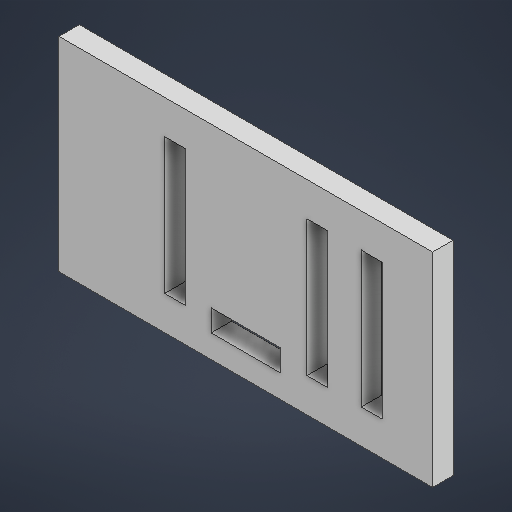
# Autodesk Inventor part: Moving_rail
Saved by Autodesk Inventor 2027 (Build 310192000, 192)
## iProperties
Created: 2026-05-09
Part Number: Moving_rail
Material: Generic
Document SubType Name: Modeling
Designer: alexy
Density: 1 g/cm^3
Appearance: Default
Mass: 3.22008 g
Surface Area: 29.3032 cm^2
Volume: 3.22008 cm^3
Author: alexy
Autodesk Inventor part; units mm, degrees
ref_plane "YZ Plane" through (0, 0, 0) normal (1, 0, 0) x (0, 1, 0)
ref_plane "XZ Plane" through (0, 0, 0) normal (0, 1, 0) x (-1, 0, 0)
ref_plane "XY Plane" through (0, 0, 0) normal (0, 0, 1) x (1, 0, 0)
sketch "Sketch1" plane through (0, 0, 0) normal (0, 0, 1) x (1, 0, 0)
  line L0 (0, 0) -> (55, 0)
  line L1 (55, 0) -> (55, 30)
  line L2 (55, 30) -> (0, 30)
  line L3 (0, 30) -> (0, 0)
  line L4 (36.5, 25) -> (39.55, 25)
  line L5 (39.55, 25) -> (39.55, 5)
  line L6 (39.55, 5) -> (36.5, 5)
  line L7 (36.5, 5) -> (36.5, 25)
  line L8 (15.55, 25) -> (18.6, 25)
  line L9 (18.6, 25) -> (18.6, 5)
  line L10 (18.6, 5) -> (15.55, 5)
  line L11 (15.55, 5) -> (15.55, 25)
  line L12 (44.5, 25) -> (47.55, 25)
  line L13 (47.55, 25) -> (47.55, 5)
  line L14 (47.55, 5) -> (44.5, 5)
  line L15 (44.5, 5) -> (44.5, 25)
  point P0 (15.55, 15)
  point P1 (0, 15)
  point P2 (36.5, 15)
  point P3 (17.075, 5)
  point P4 (27.5, 30)
  dimension "d0" = 55
  dimension "d1" = 30
  dimension "d2" = 3.05
  dimension "d3" = 3.05
  dimension "d4" = 24
  dimension "d6" = 10
  dimension "d7" = 8.9
  dimension "d16" = 3.05
  dimension "d17" = 32
  constraints: 32 end point, 8 parallel, 5 midpoint, 4 horizontal, 4 horizontal alignment, 4 perpendicular, 2 point on line
  measures "d0" distance of L2.end L1.end
  measures "d1" distance of L0.end L1.end
  measures "d2" distance of L5.end L6.end
  measures "d3" distance of L9.end L10.end
  measures "d4" distance between parallel lines of L11 L5
  measures "d6" vertical distance of point (15.55, 15) point (17.075, 5)
  measures "d7" distance from line of L9 point (27.5, 30)
  measures "d16" distance of L13.end L14.end
  measures "d17" distance of L10.end L13.end
extrude "Extrusion1" add sketch "Sketch1" along normal blind 3
sketch "Sketch2" plane through (0, 0, 3) normal (0, 0, 1) x (1, 0, 0)
  line L0 (22.4, 6.6) -> (32.6, 6.6)
  line L1 (32.6, 6.6) -> (32.6, 3.4)
  line L2 (32.6, 3.4) -> (22.4, 3.4)
  line L3 (22.4, 3.4) -> (22.4, 6.6)
  line L4 (22.4, 6.6) -> (32.6, 3.4) construction
  line L5 (32.6, 6.6) -> (22.4, 3.4) construction
  line L6 (55, 30) -> (0, 30) projected
  line L7 (0, 0) -> (55, 0) projected
  point P0 (27.5, 5)
  point P1 (27.5, 30)
  point P2 (27.5, 30)
  dimension "d11" = 3.2
  dimension "d12" = 10.2
  dimension "d15" = 5
  constraints: 12 end point, 4 midpoint, 2 parallel, 1 horizontal, 1 perpendicular, 1 vertical alignment
  measures "d11" distance of L0.end L1.end
  measures "d12" distance between parallel lines of L3 L1
  measures "d15" distance from line of L7 point (27.5, 5)
extrude "Extrusion2" cut sketch "Sketch2" against normal blind 3
body "Solid1"
